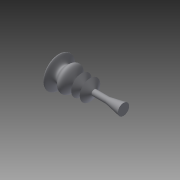
# Autodesk Inventor part: emitter
Saved by Autodesk Inventor 2015 (Build 190159000, 159)
## iProperties
Created: 2016-03-12
Part Number: emitter
Material: Generic
Document SubType Name: Modeling
Designer: Administrator
Density: 1 g/cm^3
Appearance: Default
particle.settings: {"charge":1, "dir":[1,0,0], "rate": 100, "velocity": 5, "spread": 0.09, "select":true, "transfo":true, "clr":"00B800"}
particle.name: particle.emitter
Author: Administrator
Autodesk Inventor part; units mm, degrees
ref_plane "YZ Plane" through (0, 0, 0) normal (1, 0, 0) x (0, 1, 0)
ref_plane "XZ Plane" through (0, 0, 0) normal (0, 1, 0) x (-1, 0, 0)
ref_plane "XY Plane" through (0, 0, 0) normal (0, 0, 1) x (1, 0, 0)
sketch "Sketch1" plane through (0, 0, 0) normal (0, 0, 1) x (1, 0, 0)
  line L0 (5.5321, 0) -> (-7.1679, 0)
  line L1 (5.5321, 0) -> (5.5321, 1.0691)
  line L2 (5.5321, 1.0691) -> (2.6354, 0.5346)
  line L3 (2.6354, 0.5346) -> (0, 0.5346)
  line L4 (0, 0.5346) -> (-0.8179, 1.9423)
  line L5 (-0.8179, 1.9423) -> (-1.6203, 0.5346)
  line L6 (-1.6203, 0.5346) -> (-2.4382, 1.9423)
  line L7 (-2.4382, 1.9423) -> (-3.2406, 0.5346)
  spline S0 degree 4 poles (-3.2406, 0.5346) (-3.3952, 0.0948) (-4.5705, 6.9509) (-6.3621, -4.4832) (-6.5726, 6.5277) (-7.1679, 0) knots 0 0 0 0 0 0.468838 1 1 1 1 1
  point P0 (0, 0)
  point P1 (-3.8789, 1.8233)
  point P2 (-4.7311, 2.3081)
  point P3 (-5.6803, 1.5242)
  point P4 (-6.3128, 2.2848)
  dimension "d0" = 12.7
  dimension "d1" = 1.0691
  constraints: 16 end point, 2 parallel, 2 point on line, 1 horizontal, 1 perpendicular, 1 vertical, 6 other
  measures "d0" distance of L0.start L0.end
  measures "d1" distance of L0.start L1.end
revolve "Revolution1" add sketch "Sketch1" angle 360 about axis through (5.5321, 0, 0) along (-1, 0, 0)
body "Solid1"
